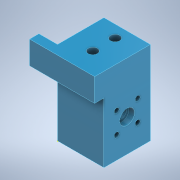
# Autodesk Inventor part: suport tija
Saved by Autodesk Inventor 2022 (Build 260153000, 153)
## iProperties
Created: 2022-03-04
Part Number: suport tija
Material: PET Plastic
Document SubType Name: Modeling
Designer: Oana
Density: 1.541 g/cm^3
Appearance: Sky Blue Dark
Author: Oana
Autodesk Inventor part; units mm, degrees
ref_plane "YZ Plane" through (0, 0, 0) normal (1, 0, 0) x (0, 1, 0)
ref_plane "XZ Plane" through (0, 0, 0) normal (0, 1, 0) x (-1, 0, 0)
ref_plane "XY Plane" through (0, 0, 0) normal (0, 0, 1) x (1, 0, 0)
sketch "Sketch1" plane through (0, 0, 0) normal (0, 1, 0) x (-1, 0, 0)
  point P0 (0, 0)
sketch "Sketch2" plane through (0, 0, 0) normal (0, 1, 0) x (-1, 0, 0)
  line L0 (0, 0) -> (-25, 0)
  line L1 (-25, 0) -> (-25, -25)
  line L2 (-25, -25) -> (0, -25)
  line L3 (0, -25) -> (0, 0)
  dimension "d0" = 25
  constraints: 8 end point, 2 parallel, 2 perpendicular, 1 horizontal
  measures "d0" distance of L2.end L0.start
extrude "Extrusion1" add sketch "Sketch2" along normal blind 35
sketch "Sketch3" plane through (25, 0, 0) normal (1, 0, 0) x (0, 0, -1)
  circle A0 centre (12.5, 17.5) radius 2.5
  line L0 (0, 0) -> (25, 0) projected
  line L1 (25, 0) -> (25, 35) projected
  line L2 (0, 35) -> (25, 35) projected
  line L3 (0, 0) -> (0, 35) projected
  line L4 (0, 35) -> (25, 0) construction
  line L5 (0, 0) -> (25, 35) construction
  line L6 (12.5, 17.5) -> (12.5, 0) construction
  point P0 (0, 0)
  dimension "d8" = 5
  constraints: 6 end point, 3 midpoint, 1 centre point, 1 coincident
  measures "d8" diameter of A0
extrude "Extrusion2" cut sketch "Sketch3" against normal through all contours A0
sketch "Sketch4" plane through (0, 35, 0) normal (0, 1, 0) x (1, 0, 0)
  line L0 (25, 0) -> (25, 25) projected
  line L1 (25, 25) -> (0, 25) projected
  line L2 (0, 25) -> (0, 0) projected
  line L3 (0, 0) -> (25, 0) projected
  line L4 (0, 25) -> (25, 0) construction
  line L5 (0, 0) -> (25, 25) construction
  line L6 (12.5, 12.5) -> (12.5, 18.5)
  line L7 (12.5, 12.5) -> (12.5, 6.5)
  circle A0 centre (12.5, 18.5) radius 2.5
  circle A1 centre (12.5, 6.5) radius 2.5
  dimension "d18" = 6
  dimension "d19" = 5
  constraints: 8 end point, 2 centre point, 2 coincident, 1 collinear, 1 equal radius, 1 midpoint, 1 perpendicular, 1 point on line, 1 vertical
  measures "d18" distance of L6.start L6.end
  measures "d19" diameter of A0
extrude "Extrusion3" cut sketch "Sketch4" against normal blind 15 contours A0 | A1
ref_plane "Work Plane1" through (25, 2, -23) normal (1, 0, 0) x (0, 0, -1)
sketch "Sketch5" plane through (25, 2, -23) normal (1, 0, 0) x (0, 0, -1)
  circle A0 centre (-16.1569, 21.1569) radius 1.35 projected
  circle A1 centre (-4.8431, 21.1569) radius 1.35 projected
  circle A2 centre (-4.8431, 9.8431) radius 1.35 projected
  circle A3 centre (-16.1569, 9.8431) radius 1.35 projected
  point P0 (-23, -2)
extrude "Extrusion4" cut sketch "Sketch5" against normal through all
sketch "Sketch7" plane through (0, 35, 0) normal (0, 1, 0) x (1, 0, 0)
  circle A0 centre (12.5, 18.5) radius 2.5 projected
  circle A1 centre (12.5, 6.5) radius 2.5 projected
  line L0 (25, 0) -> (25, 25) projected
  line L1 (25, 25) -> (0, 25) projected
  line L2 (0, 25) -> (0, 0) projected
  line L3 (0, 0) -> (25, 0) projected
extrude "Extrusion6" add sketch "Sketch7" along normal blind 10
sketch "Sketch10" plane through (0, 0, -25) normal (-1, 0, 0) x (0, 0, 1)
  point P0 (25, 0)
sketch "Sketch11" plane through (0, 0, -25) normal (-1, 0, 0) x (0, 0, 1)
  circle A0 centre (12.5, 17.5) radius 2.5 projected
  circle A1 centre (12.5, 17.5) radius 10.5
  point P0 (25, 0)
  dimension "d27" = 21
  constraints: 1 centre point, 1 coincident
  measures "d27" diameter of A1
extrude "Extrusion9" cut sketch "Sketch11" against normal blind 5
sketch "Sketch12" plane through (25, 0, 0) normal (1, 0, 0) x (0, 0, -1)
  circle A0 centre (12.5, 17.5) radius 2.5 projected
  circle A1 centre (12.5, 17.5) radius 4
  point P0 (0, 0)
  dimension "d30" = 8
  constraints: 1 centre point, 1 coincident
  measures "d30" diameter of A1
extrude "Extrusion10" cut sketch "Sketch12" against normal blind 3
sketch "Sketch13" plane through (0, 0, 0) normal (0, 0, 1) x (1, 0, 0)
  line L0 (25, 45) -> (25, 32.5) projected
  line L1 (25, 32.5) -> (-10, 32.5) projected
  line L2 (-10, 45) -> (-10, 32.5) projected
  line L3 (25, 45) -> (-10, 45) projected
  point P0 (0, 0)
extrude "Extrusion11" add sketch "Sketch13" along normal blind 5
equation "\"d0\" = lungime"
equation "\"lungime\" = 25"
equation "\"latime\" = 25"
body "Solid1"
